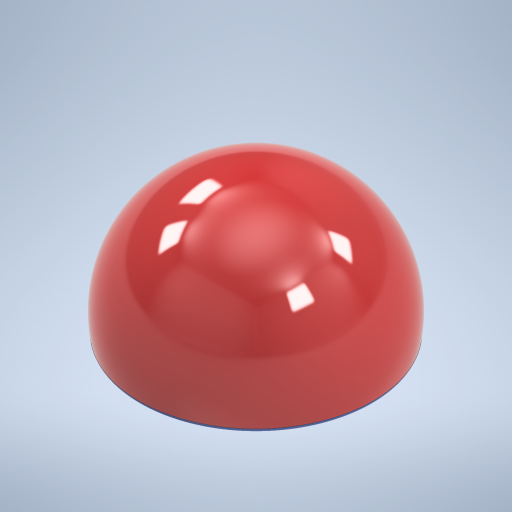
# Autodesk Inventor part: Dianecap
Saved by Autodesk Inventor 2023 (Build 270158000, 158)
## iProperties
Created: 2022-12-04
Part Number: Dianecap
Material: Generic
Document SubType Name: Modeling
Designer: holly
Density: 1 g/cm^3
Appearance: Default
Author: holly
Autodesk Inventor part; units mm, degrees
ref_plane "YZ Plane" through (0, 0, 0) normal (1, 0, 0) x (0, 1, 0)
ref_plane "XZ Plane" through (0, 0, 0) normal (0, 1, 0) x (-1, 0, 0)
ref_plane "XY Plane" through (0, 0, 0) normal (0, 0, 1) x (1, 0, 0)
sketch "Sketch1" plane through (0, 0, 0) normal (0, 0, 1) x (1, 0, 0)
  arc A0 (0, 18.5) -> (-18, -4.272) centre (0, 0) ccw
  arc A1 (0, 21) -> (-20.5609, -4.272) centre (0, 0) ccw
  line L0 (0, 21) -> (0, 18.5)
  line L1 (-18, -4.272) -> (-20.5609, -4.272)
  point P0 (0, 19.75)
  dimension "d0" = 37
  dimension "d1" = 42
  dimension "d5" = 2.5609
  dimension "d6" = 2.5
  constraints: 4 end point, 4 point on circle, 2 centre point, 2 coincident, 1 horizontal, 1 midpoint, 1 vertical
  measures "d0" diameter of A0
  measures "d1" diameter of A1
  measures "d5" distance of L1.end L1.start
  measures "d6" distance of L0.start L0.end
revolve "Revolution1" add sketch "Sketch1" angle 360 about axis through (0, 21, 0) along (0, -1, 0)
fillet "Fillet1" radius 1 2 edges at (20.5609, -4.272, 0) (18, -4.272, 0)
body "Solid1"
